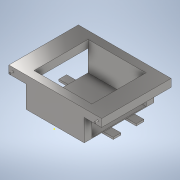
# Autodesk Inventor part: часть транспортера
Saved by Autodesk Inventor 2020.1 (Build 241239000, 239)
## iProperties
Created: 2021-10-28
Part Number: часть транспортера
Material: Железо, ковкое
Document SubType Name: Modeling
Designer: Ni3na
Density: 7.15 g/cm^3
Appearance: С умеренной полировкой
Author: Ni3na
Autodesk Inventor part; units mm, degrees
ref_plane "YZ Plane" through (0, 0, 0) normal (1, 0, 0) x (0, 1, 0)
ref_plane "XZ Plane" through (0, 0, 0) normal (0, 1, 0) x (-1, 0, 0)
ref_plane "XY Plane" through (0, 0, 0) normal (0, 0, 1) x (1, 0, 0)
sketch "Эскиз1" plane through (0, 0, 0) normal (0, 1, 0) x (-1, 0, 0)
  line L0 (100.4756, 42.2222) -> (-99.5244, 42.2222)
  line L1 (-99.5244, 42.2222) -> (-99.5244, 22.2222)
  line L2 (-99.5244, 22.2222) -> (100.4756, 22.2222)
  line L3 (100.4756, 22.2222) -> (100.4756, 42.2222)
  line L4 (101, -17.7778) -> (-99, -17.7778)
  line L5 (-99, -17.7778) -> (-99, -37.7778)
  line L6 (-99, -37.7778) -> (101, -37.7778)
  line L7 (101, -37.7778) -> (101, -17.7778)
  point P0 (0, 0)
  dimension "d0" = 200
  dimension "d1" = 20
  dimension "d2" = 200
  dimension "d3" = 20
  dimension "d4" = 40
  constraints: 16 end point, 4 parallel, 2 horizontal, 2 perpendicular
  measures "d0" distance of L1.end L2.end
  measures "d1" distance of L2.end L0.start
  measures "d2" distance of L5.end L6.end
  measures "d3" distance of L6.end L4.start
  measures "d4" distance between parallel lines of L2 L4
extrude "Выдавливание1" add sketch "Эскиз1" along normal blind 5
sketch "Эскиз2" plane through (0, 5, 0) normal (0, 1, 0) x (1, 0, 0)
  line L0 (-75.4756, -92.2222) -> (74.5244, -92.2222)
  line L1 (74.5244, -92.2222) -> (74.5244, 87.7778)
  line L2 (74.5244, 87.7778) -> (-75.4756, 87.7778)
  line L3 (-75.4756, 87.7778) -> (-75.4756, -92.2222)
  line L4 (-100.4756, -42.2222) -> (99.5244, -42.2222) projected
  line L5 (99.5244, -42.2222) -> (99.5244, -22.2222) projected
  line L6 (-100.4756, -22.2222) -> (-100.4756, -42.2222) projected
  point P0 (0, 0)
  dimension "d7" = 180
  dimension "d8" = 50
  dimension "d11" = 150
  dimension "d12" = 25
  constraints: 8 end point, 2 parallel, 1 horizontal, 1 perpendicular
  measures "d7" distance of L2.end L0.start
  measures "d8" distance between parallel lines of L0 L4
  measures "d11" distance of L1.end L2.end
  measures "d12" distance between parallel lines of L5 L1
extrude "Выдавливание2" add sketch "Эскиз2" along normal blind 2
sketch "Эскиз3" plane through (0, 7, 0) normal (0, 1, 0) x (1, 0, 0)
  line L0 (-75.4756, 87.7778) -> (-75.4756, -92.2222) projected
  line L1 (74.5244, -92.2222) -> (74.5244, 87.7778) projected
  line L2 (-75.4756, -92.2222) -> (74.5244, -92.2222)
  line L3 (74.5244, -92.2222) -> (74.5244, -72.2222)
  line L4 (74.5244, -72.2222) -> (-75.4756, -72.2222)
  line L5 (-75.4756, -72.2222) -> (-75.4756, -92.2222)
  line L6 (-75.4756, 67.6742) -> (74.5244, 67.6742)
  line L7 (74.5244, 67.6742) -> (74.5244, 87.6742)
  line L8 (74.5244, 87.6742) -> (-75.4756, 87.6742)
  line L9 (-75.4756, 87.6742) -> (-75.4756, 67.6742)
  point P0 (0, 0)
  point P1 (-75.4756, 87.6742)
  dimension "d14" = 20
  dimension "d15" = 20
  constraints: 16 end point, 4 parallel, 3 point on line, 2 horizontal, 2 perpendicular
  measures "d14" distance between parallel lines of L4 L2
  measures "d15" distance between parallel lines of L8 L6
extrude "Выдавливание3" add sketch "Эскиз3" along normal blind 75 contours L8 L1 L6 L0 | L4 L1 L2 L0
sketch "Эскиз4" plane through (74.5244, 5, 92.2222) normal (1, 0, 0) x (0, 0, -1)
  line L0 (0, 77) -> (20, 77) projected
  line L1 (179.8965, 2) -> (179.8965, 77) projected
  line L2 (0, 77) -> (179.8965, 77)
  line L3 (179.8965, 77) -> (179.8965, 57)
  line L4 (179.8965, 57) -> (0, 57)
  line L5 (0, 57) -> (0, 77)
  point P0 (92.2222, -5)
  dimension "d18" = 20
  constraints: 8 end point, 2 parallel, 1 horizontal, 1 perpendicular, 1 point on line
  measures "d18" distance between parallel lines of L2 L4
extrude "Выдавливание4" add sketch "Эскиз4" along normal blind 45
sketch "Эскиз5" plane through (-75.4756, 5, -87.7778) normal (-1, 0, 0) x (0, 0, 1)
  line L0 (0.1035, 57) -> (0.1035, 77) projected
  line L1 (180, 0) -> (180, 57) projected
  line L2 (0.1035, 77) -> (180, 77)
  line L3 (180, 77) -> (180, 57)
  line L4 (180, 57) -> (0.1035, 57)
  line L5 (0.1035, 57) -> (0.1035, 77)
  point P0 (87.7778, -5)
  constraints: 8 end point, 2 parallel, 1 horizontal, 1 perpendicular
extrude "Выдавливание5" add sketch "Эскиз5" along normal blind 45
sketch "Эскиз6" plane through (74.5244, 7, -87.6742) normal (0, 0, -1) x (-1, 0, 0)
  circle A0 centre (185, 65) radius 2.5
  line L0 (195, 75) -> (195, 55) projected
  circle A1 centre (-35, 65) radius 2.5
  line L1 (-45, 55) -> (-45, 75) projected
  line L2 (195, 75) -> (-45, 75) projected
  point P0 (74.5244, -7)
  dimension "d23" = 10
  dimension "d24" = 5
  dimension "d25" = 5
  dimension "d26" = 10
  dimension "d27" = 10
  dimension "d28" = 10
  constraints: 2 centre point
  measures "d23" distance from line of L0 A0.centre
  measures "d24" diameter of A0
  measures "d25" diameter of A1
  measures "d26" distance from line of L1 A1.centre
  measures "d27" distance from line of L2 A1.centre
  measures "d28" distance from line of L2 A0.centre
extrude "Выдавливание6" add sketch "Эскиз6" along normal blind 3
sketch "Эскиз7" plane through (-75.4756, 5, 92.2222) normal (0, 0, 1) x (1, 0, 0)
  circle A0 centre (-35, 67) radius 2.5 projected
  circle A1 centre (-35, 67) radius 2.5
  circle A2 centre (185, 67) radius 2.5 projected
  circle A3 centre (185, 67) radius 2.5
  point P0 (75.4756, -5)
  constraints: 2 centre point, 2 coincident
extrude "Выдавливание7" add sketch "Эскиз7" along normal blind 3
sketch "Эскиз8" plane through (-110.4756, 72, 95.2222) normal (0, 0, 1) x (1, 0, 0)
  point P0 (110.4756, -72)
sketch "Эскиз9" plane through (109.5244, 72, -90.6742) normal (0, 0, -1) x (-1, 0, 0)
  circle A0 centre (0, 0) radius 2.5 projected
  circle A1 centre (0, 0) radius 2.5
  circle A2 centre (220, 0) radius 2.5 projected
  circle A3 centre (220, 0) radius 2.5
  point P0 (109.5244, -72)
  constraints: 2 centre point, 2 coincident
extrude "Выдавливание8" add sketch "Эскиз9" along normal blind 4
sketch "Эскиз10" plane through (-75.4756, 5, 92.2222) normal (0, 0, 1) x (1, 0, 0)
  circle A0 centre (-35, 67) radius 2.5 projected
  circle A1 centre (-35, 67) radius 2.5
  circle A2 centre (185, 67) radius 2.5 projected
  circle A3 centre (185, 67) radius 2.5
  point P0 (75.4756, -5)
  constraints: 2 centre point, 2 coincident
extrude "Выдавливание9" add sketch "Эскиз10" along normal blind 7
